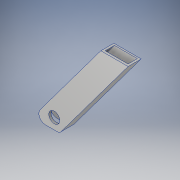
# Autodesk Inventor part: Asiento - Soporte Manija
Saved by Autodesk Inventor 2019 (Build 230136000, 136)
## iProperties
Created: 2019-11-14
Part Number: Asiento - Soporte Manija
Material: Aluminio 6061
Document SubType Name: Modeling
Designer: eddysanoli
Density: 2.7 g/cm^3
Appearance: Aluminio - Plano
Author: eddysanoli
Autodesk Inventor part; units mm, degrees
ref_plane "YZ Plane" through (0, 0, 0) normal (1, 0, 0) x (0, 1, 0)
ref_plane "XZ Plane" through (0, 0, 0) normal (0, 1, 0) x (-1, 0, 0)
ref_plane "XY Plane" through (0, 0, 0) normal (0, 0, 1) x (1, 0, 0)
sketch "Boceto1" plane through (0, 0, 0) normal (0, 1, 0) x (-1, 0, 0)
  line L0 (12.5, 6.25) -> (-12.5, 6.25)
  line L1 (-12.5, 6.25) -> (-12.5, -6.25)
  line L2 (-12.5, -6.25) -> (12.5, -6.25)
  line L3 (12.5, -6.25) -> (12.5, 6.25)
  line L4 (10.5, 4.25) -> (-10.5, 4.25)
  line L5 (-10.5, 4.25) -> (-10.5, -4.25)
  line L6 (-10.5, -4.25) -> (10.5, -4.25)
  line L7 (10.5, -4.25) -> (10.5, 4.25)
  point P0 (0, 0)
  point P1 (12.5, 0)
  point P2 (0, -6.25)
  point P3 (10.5, 0)
  point P4 (0, 4.25)
  dimension "d3" = 25
  dimension "d4" = 12.5
  dimension "d6" = 2
  dimension "d7" = 2
  constraints: 16 end point, 4 midpoint, 4 parallel, 2 horizontal, 2 horizontal alignment, 2 perpendicular, 2 vertical alignment
  measures "d3" distance between parallel lines of L1 L3
  measures "d4" distance of L2.end L0.start
  measures "d6" distance between parallel lines of L3 L7
  measures "d7" distance between parallel lines of L0 L4
sketch "Boceto2" plane through (0, 0, 0) normal (0, 0, 1) x (1, 0, 0)
  line L0 (0, 0) -> (-62.7506, -84.1864)
  line L1 (0, 0) -> (0, -34.6116) construction
  dimension "d2" = 36.7
  dimension "d5" = 105
  constraints: 4 end point, 1 vertical
  measures "d2" angle of L1 L0
  measures "d5" distance of L0.start L0.end
sweep "Barrido1" add profiles "Boceto1" path "Boceto2"
sketch "Boceto3" plane through (-12.5, 0, 6.25) normal (0, 0, 1) x (1, 0, 0)
  line L0 (0, 0) -> (25, 0) projected
  line L1 (0, 0) -> (-62.7506, -84.1864) projected
  line L2 (-37.7506, -84.1864) -> (-62.7506, -84.1864) projected
  line L3 (25, 0) -> (-37.7506, -84.1864) projected
  line L4 (25, 0) -> (-37.7506, -84.1864) projected
  line L5 (25, 0) -> (-36.551, -82.5769)
  line L6 (-37.7506, -84.1864) -> (-62.7506, -84.1864) projected
  line L7 (0, 0) -> (-62.7506, -84.1864) projected
  line L8 (-55.6056, -74.6007) -> (0, 0)
  line L9 (0, 0) -> (25, 0) projected
  line L10 (0, 0) -> (25, 0)
  line L11 (-39.7581, -84.1864) -> (-50.795, -84.1864)
  arc A0 (-39.7581, -84.1864) -> (-36.551, -82.5769) centre (-39.7581, -80.1864) ccw
  arc A1 (-55.6056, -74.6007) -> (-50.795, -84.1864) centre (-50.795, -78.1864) ccw
  line L12 (12.5, 0) -> (-50.2506, -84.1864) projected
  dimension "d10" = 4
  dimension "d11" = 6
  constraints: 8 end point, 4 collinear, 4 point on circle, 4 point on line, 4 tangent, 2 centre point
  measures "d10" radius of A0
  measures "d11" radius of A1
extrude "Extrusión1" cut sketch "Boceto3" against normal blind 12 contours L0 L12 L2 A1 L1 | L0 L3 A0 L2 L12 keep common part
sketch "Boceto4" plane through (-12.5, 0, 6.25) normal (0, 0, 1) x (1, 0, 0)
  circle A0 centre (-42.6056, -74.1864) radius 5
  line L0 (-39.7581, -84.1864) -> (-50.795, -84.1864) projected
  line L1 (0, 0) -> (-55.6056, -74.6007) projected
  point P0 (12.5, 0)
  dimension "d16" = 10
  dimension "d17" = 13
  dimension "d18" = 10
  constraints: 1 centre point
  measures "d16" distance from line of L0 A0.centre
  measures "d17" horizontal distance of L1.end A0.centre
  measures "d18" diameter of A0
extrude "Extrusión2" cut sketch "Boceto4" against normal blind 12
equation "\"d4\" = 0.5 * d3"
